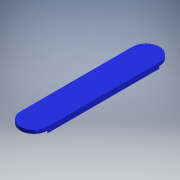
# Autodesk Inventor part: Middle_leg
Saved by Autodesk Inventor 2017 (Build 210142000, 142)
## iProperties
Part Number: Middle_leg
Material: Generic
Document SubType Name: Modeling
Designer: alex-
Appearance: Blue - Wall Paint - Glossy
Author: alex-
Autodesk Inventor part; units mm, degrees
ref_plane "YZ Plane" through (0, 0, 0) normal (1, 0, 0) x (0, 1, 0)
ref_plane "XZ Plane" through (0, 0, 0) normal (0, 1, 0) x (-1, 0, 0)
ref_plane "XY Plane" through (0, 0, 0) normal (0, 0, 1) x (1, 0, 0)
sketch "Sketch1" plane through (0, 0, 0) normal (0, 1, 0) x (-1, 0, 0)
  circle A0 centre (0, 50) radius 12 construction
  circle A1 centre (0, -50) radius 12 construction
  line L0 (0, 50) -> (0, -50) construction
  line L1 (12, 50) -> (12, -50)
  line L2 (-12, 50) -> (-12, -50)
  arc A2 (12, 50) -> (-12, 50) centre (0, 50) ccw
  arc A3 (-12, -50) -> (12, -50) centre (0, -50) ccw
  point P0 (0, 0)
  point P1 (0, 0)
  dimension "ml_length" = 100
  dimension "d1" = 24
  constraints: 8 point on circle, 6 end point, 4 centre point, 4 tangent, 2 concentric, 2 vertical alignment, 1 coincident, 1 equal radius, 1 midpoint, 1 vertical
  measures "ml_length" distance of L0.end L0.start
  measures "d1" diameter of A0
extrude "Extrusion1" add sketch "Sketch1" along normal blind 5
sketch "Sketch2" plane through (0, 0, 0) normal (0, -1, 0) x (1, 0, 0)
  circle A0 centre (0, 50) radius 12
  circle A1 centre (0, -50) radius 12
  arc A2 (12, 50) -> (-12, 50) centre (0, 50) ccw projected
  arc A3 (-12, -50) -> (12, -50) centre (0, -50) ccw projected
  point P0 (0, 0)
  constraints: 4 concentric, 2 centre point
extrude "Extrusion2" cut sketch "Sketch2" against normal blind 2
equation "\"d1\" = sa_diameter"
equation "\"d2\" = b_mat_thickness"
equation "\"d4\" = sa_thickness"
equation "\"sa_diameter\" = 24"
equation "\"b_mat_thickness\" = 5"
equation "\"sa_thickness\" = 2"
body "Solid1"
